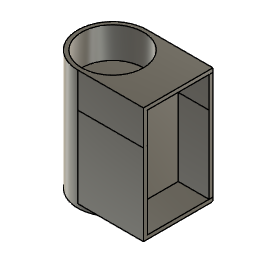
Motor Lid & Electrical housing v1 (Autodesk Fusion 360 design; units mm, degrees)
Autodesk Fusion 360 part; units mm, degrees
sketch "Sketch1" plane through (0, 0, 0) normal (0, 0, 1) x (1, 0, 0)
  circle A0 centre (0, 0) radius 50.8
  circle A1 centre (0, 0) radius 57.15
  dimension "d1" = 101.6
  dimension "d2" = 114.3
  constraint coincident A0.centre A1.centre
  measures "d1" diameter of A0
  measures "d2" diameter of A1
extrude "Extrude1" add sketch "Sketch1" along normal blind 6.35
sketch "Sketch2" plane through (0, 0, 6.35) normal (0, 0, 1) x (-1, 0, 0)
  circle A0 centre (0, 0) radius 50.8
  circle A1 centre (0, 0) radius 57.15
  circle A2 centre (0, 0) radius 50.8
  circle A3 centre (0, 0) radius 57.15
  line L0 (0, 57.15) -> (0, -57.15)
  line L1 (0, -57.15) -> (-57.15, -57.15)
  line L2 (-57.15, -57.15) -> (-57.15, 57.15)
  line L3 (-57.15, 57.15) -> (0, 57.15)
  line L4 (-57.15, -57.15) -> (-57.15, 57.15)
  line L5 (-57.15, 57.15) -> (-107.95, 57.15)
  line L6 (-107.95, 57.15) -> (-107.95, -57.15)
  line L7 (-107.95, -57.15) -> (-57.15, -57.15)
  dimension "d5" = 50.8
  constraint concentric A0 A2
  constraint concentric A2 A3
  constraint perpendicular L0 L1
  constraint parallel L0 L2
  constraint parallel L1 L3
  constraint coincident A3 L0.end
  constraint vertical L0
  constraint coincident A3 L0.start
  constraint perpendicular L4 L5
  constraint parallel L4 L6
  constraint parallel L5 L7
  measures "d5" distance of L1.end L6.end
extrude "Extrude2" add sketch "Sketch2" along normal blind 6.35 contours A0 A1 A2 A3 L0 | A0 A1 A2 A3 L0 | A1 A3 L2 L3 L4 | A1 A3 L1 L2 L4 | L2 L4 L5 L6 L7
sketch "Sketch3" plane through (0, 0, 12.7) normal (0, 0, 1) x (-1, 0, 0)
  circle A0 centre (0, 0) radius 50.8
  line L0 (0, 57.15) -> (-107.95, 57.15)
  line L1 (-107.95, 57.15) -> (-107.95, -57.15)
  line L2 (-107.95, -57.15) -> (-0.0051, -57.15)
  arc A1 (-0.0051, -57.15) -> (0, 57.15) centre (0, 0) ccw
  circle A2 centre (0, 0) radius 50.8
  circle A3 centre (0, 0) radius 57.15
  line L3 (0, 0) -> (0, -50.8)
  line L4 (0, 0) -> (0, 50.8)
  line L5 (0, 50.8) -> (-107.95, 50.8)
  line L6 (0, -50.8) -> (-107.95, -50.8)
  line L7 (-0.0051, -57.15) -> (-107.95, -57.15)
  line L8 (-107.95, -50.8) -> (-107.95, -57.15)
  line L9 (0, 57.15) -> (-107.95, 57.15)
  line L10 (-107.95, 50.8) -> (-107.95, 57.15)
  line L11 (0, 0) -> (-57.15, 0)
  line L12 (-57.15, 0) -> (-57.15, -50.8)
  line L13 (-57.15, 0) -> (-57.15, 50.8)
  dimension "d8" = 50.8
  dimension "d9" = 50.8
  constraint concentric A0 A2
  constraint concentric A2 A3
  constraint coincident L2.end A3
  constraint vertical L3
  constraint coincident A0.centre A1.centre
  constraint vertical L4
  constraint coincident L1 L5.end
  constraint tangent A2 L5
  constraint perpendicular L1 L5
  constraint coincident L1 L6.end
  constraint tangent A2 L6
  constraint perpendicular L1 L6
  constraint coincident L2.end A1.start
  constraint coincident L1.end L2.start
  constraint coincident L0.start A1.end
  constraint coincident L0.end L1.start
  constraint coincident A3 L11.end
  constraint perpendicular L4 L11
  constraint coincident L6 L12.end
  constraint tangent A3 L12
  constraint coincident L5 L13.end
  constraint tangent A3 L13
  measures "d8" distance of A0.centre L3.end
  measures "d9" distance of A0.centre L4.end
extrude "Extrude3" add sketch "Sketch3" along normal blind 127 contours A0 A1 A2 A3 L5 L6 | A0 A2 A3 L5 L11 | A0 A2 A3 L6 L11 | L0 L1 A3 L5 L9 L10 | A3 L5 L13 | A3 L6 L12 | L1 L2 A3 L6 L7 L8
sketch "Sketch4" plane through (0, 0, 139.7) normal (0, 0, 1) x (-1, 0, 0)
  circle A0 centre (0, 0) radius 50.8
  line L0 (-57.15, -50.8) -> (-107.95, -50.8)
  line L1 (-107.95, -50.8) -> (-107.95, -57.15)
  line L2 (-107.95, -57.15) -> (-0.0051, -57.15)
  arc A1 (-0.0051, -57.15) -> (0, 57.15) centre (0, 0) ccw
  line L3 (0, 57.15) -> (-107.95, 57.15)
  line L4 (-107.95, 57.15) -> (-107.95, 50.8)
  line L5 (-107.95, 50.8) -> (-57.15, 50.8)
  line L6 (-57.15, 50.8) -> (-57.15, -50.8)
  circle A2 centre (0, 0) radius 6.35
  circle A3 centre (0, 0) radius 57.15
  line L7 (-0.0051, -57.15) -> (-107.95, -57.15)
  line L8 (0, 57.15) -> (-107.95, 57.15)
  line L9 (-107.95, 57.15) -> (-107.95, 50.8)
  line L10 (-107.95, 50.8) -> (-57.15, 50.8)
  line L11 (-57.15, -50.8) -> (-57.15, 50.8)
  line L12 (-57.15, -50.8) -> (-107.95, -50.8)
  line L13 (-107.95, -50.8) -> (-107.95, -57.15)
  dimension "d12" = 12.7
  constraint concentric A0 A2
  constraint concentric A2 A3
  constraint coincident L2.end A3
  constraint coincident L2.end A1.start
  constraint coincident L1.end L2.start
  constraint coincident A1.end L3.start
  constraint coincident L3.end L4.start
  constraint coincident L4.end L5.start
  constraint coincident L5.end L6.start
  constraint coincident L0.start L6.end
  constraint coincident L0.end L1.start
  measures "d12" diameter of A2
extrude "Extrude4" add sketch "Sketch4" along normal blind 6.35 contours A0 | L0 L1 L2 L6 A3 L7 L11 L12 L13 | L3 L4 L5 L6 A3 L8 L9 L10 L11 | A1 A3
sketch "Sketch5" plane through (0, 0, 146.05) normal (0, 0, 1) x (-1, 0, 0)
  circle A0 centre (0, 0) radius 6.35
  line L0 (-57.15, -50.8) -> (-107.95, -50.8)
  line L1 (-107.95, -50.8) -> (-107.95, -57.15)
  line L2 (-107.95, -57.15) -> (-0.0051, -57.15)
  arc A1 (-0.0051, -57.15) -> (0, 57.15) centre (0, 0) ccw
  line L3 (0, 57.15) -> (-107.95, 57.15)
  line L4 (-107.95, 57.15) -> (-107.95, 50.8)
  line L5 (-107.95, 50.8) -> (-57.15, 50.8)
  line L6 (-57.15, 50.8) -> (-57.15, -50.8)
  circle A2 centre (0, 0) radius 57.15
  circle A3 centre (0, 0) radius 50.8
  line L7 (-0.0051, -57.15) -> (-107.95, -57.15)
  line L8 (-107.95, -57.15) -> (-107.95, -50.8)
  line L9 (-107.95, -50.8) -> (-57.15, -50.8)
  line L10 (-57.15, -50.8) -> (-57.15, 50.8)
  line L11 (-57.15, 50.8) -> (-107.95, 50.8)
  line L12 (-107.95, 50.8) -> (-107.95, 57.15)
  line L13 (-107.95, 57.15) -> (0, 57.15)
  dimension "d15" = 101.6
  constraint coincident A0.centre A1.centre
  constraint coincident L2.end A2
  constraint concentric A2 A3
  constraint coincident L2.end A1.start
  constraint coincident L1.end L2.start
  constraint coincident L0.end L1.start
  constraint coincident L0.start L6.end
  constraint coincident L5.end L6.start
  constraint coincident L4.end L5.start
  constraint coincident L3.end L4.start
  constraint coincident A1.end L3.start
  measures "d15" diameter of A3
extrude "Extrude5" add sketch "Sketch5" along normal blind 44.45 contours L0 L1 L2 L6 A2 L7 L8 L9 L10 | L3 L4 L5 L6 A2 L10 L11 L12 L13 | A1 A2
sketch "Sketch6" plane through (57.15, 0, 0) normal (1, 0, 0) x (0, 1, 0)
  line L0 (-50.8, 12.7) -> (50.8, 12.7)
  line L1 (50.8, 12.7) -> (50.8, 139.7)
  line L2 (50.8, 139.7) -> (50.8, 190.5)
  line L3 (50.8, 190.5) -> (-50.8, 190.5)
  line L4 (-50.8, 190.5) -> (-50.8, 139.7)
  line L5 (-50.8, 139.7) -> (-50.8, 12.7)
  line L6 (0, 190.5) -> (0, 189.865)
  circle A0 centre (0, 183.515) radius 6.35
  dimension "d18" = 0.635
  dimension "d19" = 12.7
  constraint midpoint L3 L6.start
  constraint perpendicular L3 L6
  constraint coincident L6.end A0
  measures "d18" distance of L6.start L6.end
  measures "d19" diameter of A0
hole "Hole1" at (57.15, 0, 183.515) direction (-1, 0, 0) diameter 8.89 depth 8.89 tip angle 118
sketch "Sketch7" plane through (0, 0, 190.5) normal (0, 0, 1) x (-1, 0, 0)
  circle A0 centre (0, 0) radius 50.8
  arc A1 (-0.0051, -57.15) -> (0, 57.15) centre (0, 0) ccw
  line L0 (0, 57.15) -> (-107.95, 57.15)
  line L1 (-107.95, 57.15) -> (-107.95, 50.8)
  line L2 (-107.95, 50.8) -> (-57.15, 50.8)
  line L3 (-57.15, 50.8) -> (-57.15, -50.8)
  line L4 (-57.15, -50.8) -> (-107.95, -50.8)
  line L5 (-107.95, -50.8) -> (-107.95, -57.15)
  line L6 (-107.95, -57.15) -> (-0.0051, -57.15)
  circle A2 centre (0, 0) radius 50.8
  circle A3 centre (0, 0) radius 57.15
  line L7 (-0.0051, -57.15) -> (-107.95, -57.15)
  line L8 (-107.95, 57.15) -> (-107.95, -57.15)
  line L9 (-107.95, 57.15) -> (0, 57.15)
  constraint concentric A0 A2
  constraint concentric A2 A3
  constraint coincident A1.start A3
  constraint coincident A1.start L6.end
  constraint coincident L5.end L6.start
  constraint coincident L0.end L1.start
  constraint coincident A1.end L0.start
extrude "Extrude6" add sketch "Sketch7" along normal blind 6.35
